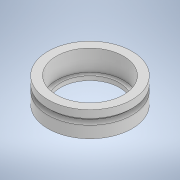
# Autodesk Inventor part: Straigthener Sleeve
Saved by Autodesk Inventor 2022.2 (Build 262287000, 287)
## iProperties
Created: 2022-08-08
Part Number: Straigthener Sleeve
Material: Generic
Document SubType Name: Modeling
Designer: Ilewicz
Density: 1 g/cm^3
Appearance: Default
Author: Ilewicz
Autodesk Inventor part; units mm, degrees
ref_plane "YZ Plane" through (0, 0, 0) normal (1, 0, 0) x (0, 1, 0)
ref_plane "XZ Plane" through (0, 0, 0) normal (0, 1, 0) x (-1, 0, 0)
ref_plane "XY Plane" through (0, 0, 0) normal (0, 0, 1) x (1, 0, 0)
sketch "Sketch2" plane through (0, 0, 0) normal (0, 0, 1) x (1, 0, 0)
  line L0 (0, -7.3481) -> (0, 7.3481) construction
  line L1 (7, 0) -> (7, 1)
  line L2 (7, 1) -> (8, 1)
  line L3 (8, 1) -> (8, 6)
  line L4 (8, 6) -> (10, 6)
  line L5 (10, 6) -> (10, 4.2071)
  line L6 (10, 4.2071) -> (9.2929, 3.5)
  line L7 (9.2929, 3.5) -> (10, 2.7929)
  line L8 (10, 2.7929) -> (10, 0)
  line L9 (10, 0) -> (7, 0)
  line L10 (8, 3.5) -> (18.2259, 3.5) construction
  circle A0 centre (10, 3.5) radius 0.5 construction
  line L11 (-3.6452, 0) -> (21.8711, 0) construction
  point P0 (0, 0)
  point P1 (0, 0)
  dimension "d1" = 1
  dimension "d2" = 1
  dimension "d3" = 5
  dimension "d4" = 1
  dimension "d5" = 8
  dimension "d6" = 2
  dimension "d7" = 2
  constraints: 22 end point, 4 vertical, 3 perpendicular, 2 collinear, 2 horizontal, 2 midpoint, 2 point on line, 1 centre point, 1 coincident, 1 tangent
  measures "d1" distance of L1.end L2.end
  measures "d2" distance of L1.start L1.end
  measures "d3" distance of L2.end L3.end
  measures "d4" diameter of A0
  measures "d5" distance between parallel lines of L0 L3
  measures "d6" distance from line of L3 A0.centre
  measures "d7" distance of L3.end L4.end
revolve "Revolution1" add sketch "Sketch2" angle 360 about axis through (0, -7.3481, 0) along (0, 1, 0)
body "Solid1"
